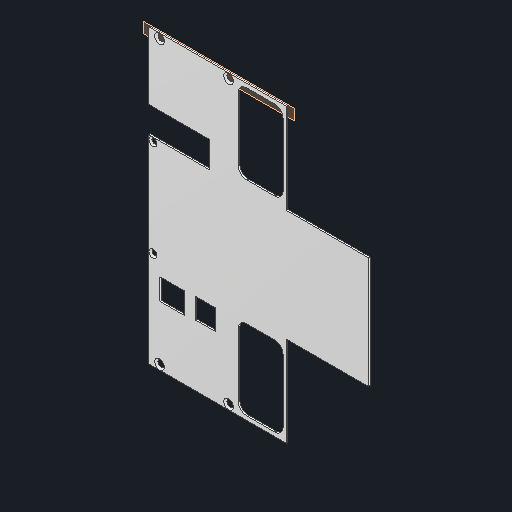
# Autodesk Inventor part: ceil
Saved by Autodesk Inventor 2023 (Build 270158000, 158)
## iProperties
Created: 2024-05-08
Part Number: ceil
Material: ABS Plastic
Document SubType Name: Modeling
Designer: szymo
Density: 1.06 g/cm^3
Appearance: Smooth - White
Mass: 15.5337 g
Surface Area: 305.16 cm^2
Volume: 14.6544 cm^3
Author: szymo
Autodesk Inventor part; units mm, degrees
ref_plane "YZ Plane" through (0, 0, 0) normal (1, 0, 0) x (0, 1, 0)
ref_plane "XZ Plane" through (0, 0, 0) normal (0, 1, 0) x (-1, 0, 0)
ref_plane "XY Plane" through (0, 0, 0) normal (0, 0, 1) x (1, 0, 0)
ref_plane "Work Plane1" through (0, 0, 0) normal (0, 0, 1) x (1, 0, 0)
sketch "Sketch1" plane through (0, 0, 0) normal (0, 0, 1) x (1, 0, 0)
  line L0 (-42, -2) -> (-73.5901, -2) projected
  arc A0 (-39.1716, -4) -> (-42, -2) centre (-42, -5) ccw projected
  arc A1 (-39.1716, -4) -> (-36.3431, -6) centre (-36.3431, -3) ccw projected
  line L1 (-36, -6) -> (-36.3431, -6) projected
  arc A2 (-36, -6) -> (-33.1612, -3.9702) centre (-36, -3) ccw projected
  line L2 (-33, -2.5071) -> (-33, -2) projected
  line L3 (-32, -1) -> (0, -1) projected
  line L4 (0, 0) -> (0, -1) projected
  line L5 (-83.8327, 0) -> (0, 0) projected
  line L6 (-83.8327, 0) -> (-83.8327, -6) projected
  line L7 (-77.8327, -6) -> (-83.8327, -6) projected
  line L8 (-41.75, -176) -> (-73.5901, -176) projected
  line L9 (-77.8327, -172) -> (-83.8327, -172) projected
  line L10 (-83.8327, -178) -> (-83.8327, -172) projected
  line L11 (-83.8327, -178) -> (0, -178) projected
  line L12 (0, -178) -> (0, -177) projected
  line L13 (-31.75, -177) -> (0, -177) projected
  line L14 (-32.75, -175) -> (-32.75, -176) projected
  arc A3 (-32.75, -175) -> (-35.75, -172) centre (-35.75, -175) ccw projected
  line L15 (-35.75, -172) -> (-36.0931, -172) projected
  arc A4 (-36.0931, -172) -> (-38.9216, -174) centre (-36.0931, -175) ccw projected
  arc A5 (-41.75, -176) -> (-38.9216, -174) centre (-41.75, -173) ccw projected
  line L16 (0, 0) -> (-83.8327, 0)
  line L17 (-83.8327, 0) -> (-83.8327, -178)
  line L18 (-83.8327, -178) -> (0, -178)
  line L19 (0, -178) -> (0, 0)
  circle A6 centre (9.325, -58.5) radius 3 projected
  line L20 (-30.35, -55) -> (-30.35, -62) projected
  line L21 (-30.35, -62) -> (50, -62) projected
  line L22 (50, -62) -> (50, -55) projected
  line L23 (50, -55) -> (-30.35, -55) projected
  circle A7 centre (-81.3327, -118.5) radius 1.75 projected
  line L24 (50, -123) -> (-83.8327, -123) projected
  line L25 (50, -116) -> (50, -123) projected
  line L26 (-30.55, -116) -> (50, -116) projected
  line L27 (-30.55, -116) -> (-30.55, -121) projected
  line L28 (-30.55, -121) -> (-46.95, -121) projected
  line L29 (-46.95, -121) -> (-46.95, -116) projected
  line L30 (-83.8327, -116) -> (-46.95, -116) projected
  line L31 (-83.8327, -123) -> (-83.8327, -116) projected
  circle A8 centre (9.325, -119.5) radius 3 projected
  line L32 (0, -55) -> (50, -55)
  line L33 (50, -55) -> (50, -123)
  line L34 (50, -123) -> (0, -123)
  line L35 (0, -123) -> (0, -55)
  arc A9 (-32, -1) -> (-33, -2) centre (-32, -2) ccw projected
  circle A10 centre (-80.8327, -3) radius 2.3 projected
  arc A11 (-73.5901, -2) -> (-77.8327, -6) centre (-73.5901, -6.25) ccw projected
  arc A12 (-33, -2.5071) -> (-33.1612, -3.9702) centre (-35.2466, -3) ccw projected
  arc A13 (-32.75, -176) -> (-31.75, -177) centre (-31.75, -176) ccw projected
  circle A14 centre (-35.2466, -175) radius 2.3 projected
  circle A15 centre (-80.8327, -175) radius 2.3 projected
  arc A16 (-77.8327, -172) -> (-73.5901, -176) centre (-73.5901, -171.75) ccw projected
  point P0 (0, -123)
  constraints: 16 end point, 4 parallel, 2 horizontal, 2 perpendicular, 2 point on line
extrude "Extrusion1" add sketch "Sketch1" along normal blind 1 contours A0 A1 L1 A2 A12 L2 A9 L3 L19 L23 L20 L21 L26 L27 L28 L29 L30 L17 L7 A11 L0 | L0 A11 L7 L6 L5 L4 L3 A9 L2 A12 A2 L1 A1 A0 | L30 L29 L28 L27 L26 L19 L24 L17 | L24 L19 L13 A13 L14 A3 L15 A4 A5 L8 A16 L9 L17 | L9 A16 L8 A5 A4 L15 A3 L14 A13 L13 L12 L11 L10 | L19 L26 L25 L24 | L23 L22 L21 L19 | L19 L21 L20 L23 | L19 L21 L33 L26 | A6 | A7 | A8 | A10 | A14 | A15
sketch "Sketch3" plane through (0, 0, 1) normal (0, 0, 1) x (1, 0, 0)
  circle A0 centre (-81.3327, -59.5) radius 1.75 projected
  circle A1 centre (-81.3327, -118.5) radius 1.75 projected
  circle A2 centre (-77.3327, -3) radius 2.3 projected
  circle A3 centre (-35.2466, -3) radius 2.3 projected
  circle A4 centre (-35.2466, -175) radius 2.3 projected
  circle A5 centre (-77.3327, -175) radius 2.3 projected
  point P0 (0, 0)
  constraints: 4 coincident
hole "Hole1" at (-35.2466, -3, 1) at (-77.3327, -3, 1) at (-77.3327, -175, 1) at (-35.2466, -175, 1) direction (0, 0, -1) diameter 3.6 end through all countersink diameter 6 countersink angle 90 clearance for "Countersunk Flat Head Screw ISO 2009/7046" size "M3" standard "ISO"
sketch "Sketch4" plane through (0, 0, 1) normal (0, 0, 1) x (1, 0, 0)
  circle A0 centre (-81.3327, -59.5) radius 1.75 projected
  circle A1 centre (-81.3327, -118.5) radius 1.75 projected
  point P0 (0, 0)
  constraints: 2 coincident
hole "Hole2" at (-81.3327, -59.5, 1) at (-81.3327, -118.5, 1) direction (0, 0, -1) diameter 3.1 end through all countersink diameter 5 countersink angle 90 clearance for "Countersunk Flat Head Screw ISO 2009/7046" size "M2.5" standard "ISO"
sketch "Sketch5" plane through (0, 0, 1) normal (0, 0, 1) x (1, 0, 0)
  line L0 (-54.55, -139.6) -> (-54.55, -129.1) projected
  line L1 (-44.05, -129.1) -> (-54.55, -129.1) projected
  line L2 (-44.05, -129.1) -> (-44.05, -139.6) projected
  line L3 (-54.55, -139.6) -> (-44.05, -139.6) projected
  line L4 (-76.05, -140.6) -> (-76.05, -129.6) projected
  line L5 (-76.05, -129.6) -> (-63.05, -129.6) projected
  line L6 (-63.05, -129.6) -> (-63.05, -140.6) projected
  line L7 (-63.05, -140.6) -> (-76.05, -140.6) projected
  line L8 (-77.05, -123) -> (-77.05, -141.6) projected
  line L9 (-77.05, -141.6) -> (-35.75, -141.6) projected
  line L10 (-35.75, -141.6) -> (-35.75, -123) projected
  line L11 (-35.75, -123) -> (-77.05, -123) projected
  circle A0 centre (-73.6, -126.3) radius 1.5 projected
  circle A1 centre (-39.2, -126.3) radius 1.5 projected
  line L12 (-68.4939, -42.5) -> (-68.4939, -56.8) projected
  line L13 (-48.1, -42.4061) -> (-68.4, -42.4061) projected
  line L14 (-47.9, -56.9) -> (-47.9, -42.4) projected
  line L15 (-68.4, -56.8939) -> (-48.1, -56.8939) projected
  line L16 (-68.8327, -42) -> (-68.8327, -57) projected
  line L17 (-83.8327, -42) -> (-68.8327, -42) projected
  line L18 (-83.8327, -57) -> (-83.8327, -42) projected
  line L19 (-68.8327, -57) -> (-83.8327, -57) projected
  line L20 (-46.9, -41) -> (-83.8327, -41)
  line L21 (-83.8327, -41) -> (-83.8327, -57)
  line L22 (-83.8327, -57) -> (-46.9, -57)
  line L23 (-46.9, -57) -> (-46.9, -41)
  line L24 (50, -123) -> (50, -55) projected
  line L25 (50, -55) -> (0, -55) projected
  line L26 (0, -55) -> (0, 0) projected
  line L27 (0, 0) -> (-35.2466, 0) projected
  circle A2 centre (-35.2466, -3) radius 3 projected
  line L28 (-35.2466, 0) -> (-77.3327, 0) projected
  circle A3 centre (-77.3327, -3) radius 3 projected
  line L29 (-77.3327, 0) -> (-83.8327, 0) projected
  line L30 (-83.8327, 0) -> (-83.8327, -59.5) projected
  circle A4 centre (-81.3327, -59.5) radius 2.5 projected
  line L31 (-83.8327, -59.5) -> (-83.8327, -118.5) projected
  circle A5 centre (-81.3327, -118.5) radius 2.5 projected
  line L32 (-83.8327, -118.5) -> (-83.8327, -178) projected
  line L33 (-83.8327, -178) -> (-77.3327, -178) projected
  circle A6 centre (-77.3327, -175) radius 3 projected
  line L34 (-77.3327, -178) -> (-35.2466, -178) projected
  circle A7 centre (-35.2466, -175) radius 3 projected
  line L35 (-35.2466, -178) -> (0, -178) projected
  line L36 (0, -178) -> (0, -123) projected
  line L37 (0, -123) -> (50, -123) projected
  line L38 (-43.05, -140.6) -> (-43.05, -128.1)
  line L39 (-43.05, -128.1) -> (-55.55, -128.1)
  line L40 (-55.55, -128.1) -> (-55.55, -140.6)
  line L41 (-55.55, -140.6) -> (-43.05, -140.6)
  line L42 (-62.05, -141.6) -> (-62.05, -128.6)
  line L43 (-62.05, -128.6) -> (-77.05, -128.6)
  line L44 (-77.05, -128.6) -> (-77.05, -141.6)
  line L45 (-77.05, -141.6) -> (-62.05, -141.6)
  line L46 (-30, -4.4) -> (-2, -4.4) projected
  line L47 (-2, -173.6) -> (-30, -173.6) projected
  line L48 (-2, -4.4) -> (-29.4, -4.4)
  line L49 (-29.4, -4.4) -> (-29.4, -2.4)
  line L50 (-29.4, -2.4) -> (-2, -2.4)
  line L51 (-2, -2.4) -> (-2, -4.4)
  line L52 (-2, -173.6) -> (-29.4, -173.6)
  line L53 (-29.4, -173.6) -> (-29.4, -175.6)
  line L54 (-29.4, -175.6) -> (-2, -175.6)
  line L55 (-2, -175.6) -> (-2, -173.6)
  line L56 (-30, -51) -> (-2, -51) projected
  line L57 (-30, -4.4) -> (-2, -4.4) projected
  line L58 (50, -123) -> (50, -55) projected
  line L59 (50, -89) -> (-83.8327, -89) construction
  line L60 (-83.8327, 0) -> (-83.8327, -178) projected
  line L61 (-2, -51) -> (-29.4, -51)
  line L62 (-29.4, -51) -> (-29.4, -2.4)
  line L63 (-29.4, -2.4) -> (-2, -2.4)
  line L64 (-2, -2.4) -> (-2, -51)
  line L65 (-30, -127) -> (-2, -127)
  line L66 (-30, -173.6) -> (-2, -173.6)
  line L67 (-29.4, -127) -> (-29.4, -175.6)
  line L68 (-29.4, -175.6) -> (-2, -175.6)
  line L69 (-2, -175.6) -> (-2, -127)
  point P0 (-29.4, -4.4)
  point P1 (-29.4, -127)
  point P2 (-2, -173.6)
  point P3 (-2, -4.4)
  point P4 (-29.4, -4.4)
  point P5 (-29.4, -51)
  dimension "d16" = 1
  dimension "d17" = 0
  dimension "d18" = 0
  dimension "d19" = 1
  dimension "d20" = 1
  dimension "d21" = 1
  dimension "d28" = 2
  dimension "d29" = 2
  constraints: 60 end point, 8 parallel, 4 horizontal, 4 perpendicular, 4 symmetric about line, 4 vertical alignment, 2 horizontal alignment, 1 midpoint, 1 point on line, 8 other
  measures "d16" distance between parallel lines of L20 L17
  measures "d17" distance between parallel lines of L19 L22
  measures "d18" distance between parallel lines of L18 L21
  measures "d19" distance between parallel lines of L23 L14
  measures "d20" distance between parallel lines of L2 L38
  measures "d21" distance between parallel lines of L6 L42
  measures "d28" distance of L48.end L49.end
  measures "d29" distance of L53.end L52.end
extrude "Extrusion2" cut sketch "Sketch5" against normal up to next contours L0 L1 L2 L3 | L4 L5 L6 L7 | L43 L42 L9 L8 | L17 L21 L20 L23 L22 L16 | L16 L19 L18 L17 | L41 L40 L39 L38 | L49 L50 L51 L46 | L46 L64 L56 L62 | L55 L54 L53 L47 | L47 L67 L65 L69
fillet "Fillet1" radius 5 8 edges at (-2, -2.4, 0.5) (-2, -51, 0.5) (-29.4, -51, 0.5) (-29.4, -2.4, 0.5) (-29.4, -127, 0.5) (-2, -175.6, 0.5) (-2, -127, 0.5) (-29.4, -175.6, 0.5)
body "Solid1"
